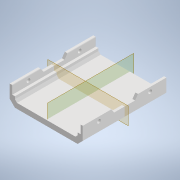
# Autodesk Inventor part: A-02
Saved by Autodesk Inventor 2022.2 (Build 262287000, 287)
## iProperties
Created: 2021-12-01
Part Number: A-02
Material: Generic
Document SubType Name: Modeling
Designer: kfcs7
Density: 1 g/cm^3
Appearance: Default
Author: kfcs7
Autodesk Inventor part; units mm, degrees
ref_plane "YZ Plane" through (0, 0, 0) normal (1, 0, 0) x (0, 1, 0)
ref_plane "XZ Plane" through (0, 0, 0) normal (0, 1, 0) x (-1, 0, 0)
ref_plane "XY Plane" through (0, 0, 0) normal (0, 0, 1) x (1, 0, 0)
sketch "Sketch1" plane through (0, 0, 0) normal (0, 1, 0) x (-1, 0, 0)
  line L0 (35, 40) -> (-35, 40)
  line L1 (-35, 40) -> (-35, -40)
  line L2 (-35, -40) -> (35, -40)
  line L3 (35, -40) -> (35, 40)
  line L4 (35, 40) -> (-35, -40) construction
  line L5 (-35, 40) -> (35, -40) construction
  point P0 (0, 0)
  dimension "d0" = 70
  dimension "d1" = 80
  constraints: 12 end point, 2 midpoint, 2 parallel, 1 horizontal, 1 perpendicular
  measures "d0" distance of L2.end L1.end
  measures "d1" distance of L1.end L0.end
extrude "Extrusion1" add sketch "Sketch1" along normal blind 17.5
chamfer "Chamfer1" distance 5 angle 45 2 edges at (35, 0, 0) (-35, 0, 0)
shell "Shell1" thickness 5 removed faces 3 at (10, 11.6667, 40) at (-10, 11.6667, -40) at (11.6667, 17.5, 13.3333)
ref_plane "Work Plane1" through (0, 17.5, -40) normal (-1, 0, 0) x (0, 0, 1)
ref_plane "Work Plane2" through (-30, 0, 0) normal (0, 0, 1) x (1, 0, 0)
sketch "Sketch6" plane through (30, 17.5, 40) normal (1, 0, 0) x (0, 0, -1)
  line L0 (80, -12.5) -> (0, -12.5) projected
  line L1 (80, -12.5) -> (80, 0) projected
  line L2 (0, 0) -> (80, 0) projected
  line L3 (0, -12.5) -> (0, 0) projected
  line L4 (0, 0) -> (0, -10.4289) projected
  line L5 (0, -8) -> (80, -8)
  point P0 (40, -17.5)
  dimension "d31" = 8
  constraints: 2 end point, 2 point on line, 1 perpendicular
  measures "d31" distance between parallel lines of L2 L5
extrude "Extrusion6" cut sketch "Sketch6" along normal blind 2.5 contours L5 L3 L2 L1
sketch "Sketch11" plane through (35, 17.5, 40) normal (1, 0, 0) x (0, 0, -1)
  line L0 (0, 9) -> (16.2241, 9) projected
  line L1 (0, 9) -> (0, 0) projected
  line L2 (0, 0) -> (27.1992, 0) projected
  line L3 (27.1992, 0) -> (30, -4) projected
  line L4 (30, -4) -> (50, -4) projected
  line L5 (50, -4) -> (52.8008, 0) projected
  line L6 (52.8008, 0) -> (80, 0) projected
  line L7 (80, 9) -> (80, 0) projected
  line L8 (63.7759, 9) -> (80, 9) projected
  line L9 (63.7759, 9) -> (60, 4.5) projected
  line L10 (20, 4.5) -> (60, 4.5) projected
  line L11 (20, 4.5) -> (16.2241, 9) projected
  line L12 (52.8008, 0) -> (27.1992, 0)
  line L13 (80, 0) -> (0, 0) projected
  point P0 (40, -17.5)
  constraints: 2 end point, 1 collinear
extrude "Extrusion11" cut sketch "Sketch11" against normal up to surface (2.5 mm away) contours L12 L5 L4 L3
fillet "Fillet3" radius 0.5 4 edges at (32.5, 17.5, 26.4004) (32.5, 17.5, -26.4004) (32.5, 13.5, -40) (32.5, 13.5, 40)
mirror "Mirror3" about plane through (0, 17.5, -40) normal (-1, 0, 0) of "Extrusion6", "Fillet3", "Extrusion11"
sketch "Sketch10" plane through (35, 17.5, 40) normal (1, 0, 0) x (0, 0, -1)
  circle A0 centre (15.4979, -4) radius 1.75 projected
  circle A1 centre (64.5021, -4) radius 1.75 projected
  point P0 (40, -17.5)
extrude "Extrusion10" cut sketch "Sketch10" against normal through all
body "Solid1"
